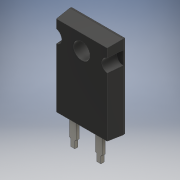
# Autodesk Inventor part: Resistor_TH-TO220
Saved by Autodesk Inventor 2018 (Build 220112000, 112)
## iProperties
Created: 2018-05-30
Part Number: Resistor_TH-TO220
Material: ABS Plastic
Document SubType Name: Modeling
Designer: Bradley
Density: 1.06 g/cm^3
Appearance: Smooth - Black
Author: Bradley
Autodesk Inventor part; units mm, degrees
ref_plane "YZ Plane" through (0, 0, 0) normal (1, 0, 0) x (0, 1, 0)
ref_plane "XY Plane" through (0, 0, 0) normal (0, 0, 1) x (1, 0, 0)
sketch "Sketch1" plane through (0, 0, 0) normal (0, 1, 0) x (-1, 0, 0)
  line L0 (5.2, -8.1) -> (-5.2, -8.1)
  line L1 (-5.2, -8.1) -> (-5.2, 8.1)
  line L2 (-5.2, 8.1) -> (5.2, 8.1)
  line L3 (5.2, 8.1) -> (5.2, -8.1)
  line L4 (5.2, -8.1) -> (-5.2, 8.1) construction
  line L5 (-5.2, -8.1) -> (5.2, 8.1) construction
  point P0 (0, 0)
  dimension "d0" = 16.2
  dimension "d1" = 10.4
  constraints: 12 end point, 2 midpoint, 2 parallel, 1 horizontal, 1 perpendicular
  measures "d0" distance of L2.end L0.start
  measures "d1" distance of L1.end L2.end
extrude "Extrusion1" add sketch "Sketch1" along normal blind 0.3 draft -5 and the other way blind 2.9 draft -5
sketch "Sketch2" plane through (0, -2.9, 0) normal (0, -1, 0) x (1, 0, 0)
  line L0 (-4.9463, -7.8463) -> (-4.9463, 7.8463) projected
  line L1 (4.9463, -7.8463) -> (-4.9463, -7.8463) projected
  line L2 (4.9463, 7.8463) -> (4.9463, -7.8463) projected
  line L3 (-4.9463, 7.8463) -> (4.9463, 7.8463) projected
  circle A0 centre (0, 4.9) radius 1.6
  line L4 (5.2, 8.1) -> (-5.2, 8.1) projected
  point P0 (0, 0)
  dimension "d6" = 3.2
  dimension "d7" = 3.2
  constraints: 1 centre point, 1 vertical alignment
  measures "d6" distance from line of A0.centre L4
  measures "d7" diameter of A0
extrude "Extrusion2" cut sketch "Sketch2" against normal through all contours A0
sketch "Sketch3" plane through (0, -2.9, 0) normal (0, -1, 0) x (1, 0, 0)
  line L0 (-4.9463, -7.8463) -> (-4.9463, 7.8463) projected
  line L1 (-5.2, 8.1) -> (-4.9463, 7.8463) projected
  line L2 (-5.2, 8.1) -> (-5.2, -8.1) projected
  line L3 (-5.2, -8.1) -> (-4.9463, -7.8463) projected
  circle A0 centre (0, 4.9) radius 1.6 projected
  line L4 (-4.9463, -7.8463) -> (-4.9463, 7.8463) projected
  line L5 (4.9463, -7.8463) -> (-4.9463, -7.8463) projected
  line L6 (4.9463, 7.8463) -> (4.9463, -7.8463) projected
  line L7 (-4.9463, 7.8463) -> (4.9463, 7.8463) projected
  line L8 (4.9463, 7.8463) -> (4.9463, -7.8463) projected
  line L9 (5.2, -8.1) -> (4.9463, -7.8463) projected
  line L10 (5.2, -8.1) -> (5.2, 8.1) projected
  line L11 (5.2, 8.1) -> (4.9463, 7.8463) projected
  line L12 (-5.2, 8.1) -> (-5.2, -8.1) projected
  arc A1 (-5.2, 3.6) -> (-5.2, 6.2) centre (-5.2, 4.9) ccw
  line L13 (5.2, -8.1) -> (5.2, 8.1) projected
  arc A2 (5.2, 6.2) -> (5.2, 3.6) centre (5.2, 4.9) ccw
  point P0 (0, 0)
  dimension "d10" = 1.3
  constraints: 6 point on line, 4 point on circle, 2 centre point, 2 horizontal alignment, 1 equal radius
  measures "d10" radius of A1
extrude "Extrusion3" cut sketch "Sketch3" against normal up to surface (2.9 mm away) contours A1 L2 L0 | L0 A1 | A2 L6 | L6 A2 L10
ref_plane "Work Plane1" through (0, -1.5, 0) normal (0, 1, 0) x (-1, 0, 0)
sketch "Sketch4" plane through (0, -1.5, 0) normal (0, 1, 0) x (-1, 0, 0)
  line L0 (-4.9463, -7.8463) -> (4.9463, -7.8463) projected
  line L1 (5.2, -8.1) -> (4.9463, -7.8463) projected
  line L2 (5.2, -8.1) -> (-5.2, -8.1) projected
  line L3 (-5.2, -8.1) -> (-4.9463, -7.8463) projected
  line L4 (3.19, -7.8463) -> (3.19, -11.563)
  line L5 (5.2, -8.1) -> (-5.2, -8.1) projected
  line L6 (3.19, -11.563) -> (3.14, -11.563)
  arc A0 (3.14, -11.563) -> (2.94, -11.763) centre (3.14, -11.763) ccw
  line L7 (2.94, -11.763) -> (2.94, -13.063)
  line L8 (2.94, -13.063) -> (2.14, -13.063)
  line L9 (2.14, -13.063) -> (2.14, -11.763)
  arc A1 (2.14, -11.763) -> (1.94, -11.563) centre (1.94, -11.763) ccw
  line L10 (1.94, -11.563) -> (1.89, -11.563)
  line L11 (1.89, -7.8463) -> (1.89, -11.563)
  circle A2 centre (0, 4.9) radius 1.6 projected
  dimension "d21" = 0.8
  dimension "d22" = 1.3
  dimension "d23" = 0.2
  dimension "d24" = 16.463
  dimension "d25" = 1.89
  dimension "d26" = 1.5
  constraints: 14 end point, 4 point on circle, 4 point on line, 3 equal length, 3 perpendicular, 3 tangent, 2 centre point, 2 parallel, 1 equal radius, 1 horizontal alignment
  measures "d21" distance between parallel lines of L9 L7
  measures "d22" distance between parallel lines of L11 L4
  measures "d23" radius of A0
  measures "d24" distance from line of A2.centre L6
  measures "d25" distance from line of L11 A2.centre
  measures "d26" distance between parallel lines of L8 L6
extrude "Extrusion4" add sketch "Sketch4" against normal blind 0.6 contours L0 L4 L2 L11 | L2 L4 L6 A0 L7 L8 L9 A1 L10 L11
mirror "Mirror1" about plane through (0, 0, 0) normal (1, 0, 0) of "Extrusion4"
sketch "Sketch5" plane through (0, 0.3, 0) normal (0, 1, 0) x (1, 0, 0)
  circle A0 centre (0, -4.9) radius 1.6 projected
  line L0 (5.1738, 8.0738) -> (5.1738, -8.0738) projected
  line L1 (-5.1738, 8.0738) -> (5.1738, 8.0738) projected
  line L2 (-5.1738, -8.0738) -> (-5.1738, 8.0738) projected
  line L3 (5.1738, -8.0738) -> (-5.1738, -8.0738) projected
  line L4 (4.25, -2.237) -> (-4.25, -2.237)
  line L5 (-4.25, -2.237) -> (-4.25, 7.163)
  line L6 (-4.25, 7.163) -> (4.25, 7.163)
  line L7 (4.25, 7.163) -> (4.25, -2.237)
  point P0 (0, 0)
  point P1 (0, -2.237)
  dimension "d34" = 8.5
  dimension "d35" = 9.4
  dimension "d36" = 2.663
  constraints: 8 end point, 2 parallel, 1 horizontal, 1 midpoint, 1 perpendicular, 1 vertical alignment
  measures "d34" distance of L4.start L4.end
  measures "d35" distance of L6.end L4.start
  measures "d36" distance from line of L4 A0.centre
extrude "Extrusion5" add sketch "Sketch5" along normal blind 0.01 contours L4 L5 L6 L7
body "Solid1"
